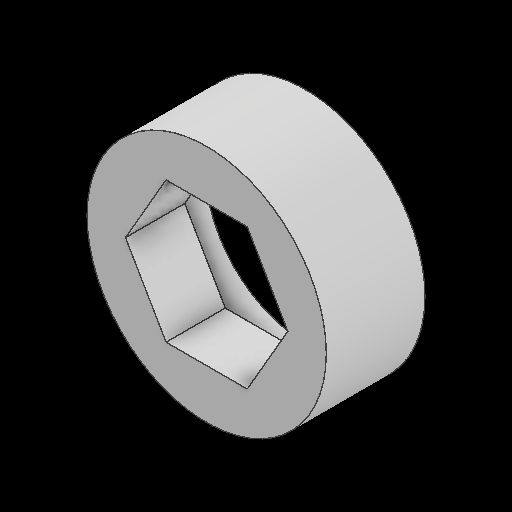
# Autodesk Inventor part: BatterySafetyCap
Saved by Autodesk Inventor 2025.2 (Build 292293000, 293)
## iProperties
Created: 2026-06-27
Part Number: BatterySafetyCap
Material: Generic
Document SubType Name: Modeling
Designer: valer
Density: 1 g/cm^3
Appearance: Default
Author: valer
Autodesk Inventor part; units mm, degrees
ref_plane "YZ Plane" through (0, 0, 0) normal (1, 0, 0) x (0, 1, 0)
ref_plane "XZ Plane" through (0, 0, 0) normal (0, 1, 0) x (-1, 0, 0)
ref_plane "XY Plane" through (0, 0, 0) normal (0, 0, 1) x (1, 0, 0)
sketch "Sketch1" plane through (0, 0, 0) normal (0, 0, 1) x (1, 0, 0)
  circle A0 centre (0, 0) radius 10.125
  circle A1 centre (0, 0) radius 12.125
  dimension "d0" = 20.25
  dimension "d1" = 2
  constraints: 2 centre point, 2 coincident
  measures "d0" diameter of A0
  measures "d1" radial gap between concentric circles of A0 A1
extrude "Extrusion1" add sketch "Sketch1" along normal blind 4
sketch "Sketch2" plane through (0, 0, 4) normal (0, 0, 1) x (1, 0, 0)
  circle A0 centre (0, 0) radius 10.125 projected
  line L0 (4.1136, 7.125) -> (8.2272, 0)
  line L1 (8.2272, 0) -> (4.1136, -7.125)
  line L2 (4.1136, -7.125) -> (-4.1136, -7.125)
  line L3 (-4.1136, -7.125) -> (-8.2272, 0)
  line L4 (-8.2272, 0) -> (-4.1136, 7.125)
  line L5 (-4.1136, 7.125) -> (4.1136, 7.125)
  line L6 (-16.975, 0) -> (16.975, 0) projected
  line L7 (0, -16.975) -> (0, 16.975) projected
  circle A1 centre (0, 0) radius 12.125 projected
  point P0 (0, 7.125)
  dimension "d4" = 14.25
  constraints: 12 end point, 1 coincident, 1 midpoint, 1 point on line, 13 other
  measures "d4" distance between parallel lines of L2 L5
extrude "Extrusion2" add sketch "Sketch2" along normal blind 6 contours L6 L0 L5 L7 A0 | L6 A1 L7 A0 | A0 L7 L2 L1 L6 | A0 L7 A1 L6 | L7 L5 L4 L6 A0 | A0 L6 A1 L7 | L7 A1 L6 A0 | A0 L6 L3 L2 L7
body "Solid1"
